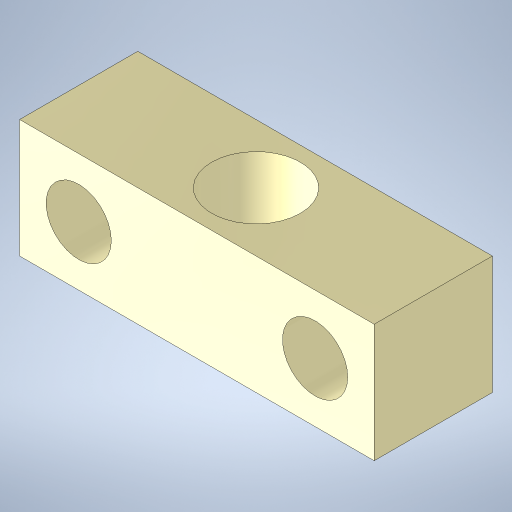
# Autodesk Inventor part: End Bushing
Saved by Autodesk Inventor 2023.2 (Build 272271000, 271)
## iProperties
Created: 2024-02-24
Part Number: End Bushing
Material: Nylon 6/6
Document SubType Name: Modeling
Designer: Nathan Cai
Density: 1.13 g/cm^3
Appearance: Nylon 6
Author: Nathan Cai
Autodesk Inventor part; units mm, degrees
ref_plane "YZ Plane" through (0, 0, 0) normal (1, 0, 0) x (0, 1, 0)
ref_plane "XZ Plane" through (0, 0, 0) normal (0, 1, 0) x (-1, 0, 0)
ref_plane "XY Plane" through (0, 0, 0) normal (0, 0, 1) x (1, 0, 0)
sketch "Sketch1" plane through (0, 0, 0) normal (0, 0, 1) x (1, 0, 0)
  line L0 (-9.525, -3.175) -> (9.525, -3.175)
  line L1 (9.525, -3.175) -> (9.525, 3.175)
  line L2 (9.525, 3.175) -> (-9.525, 3.175)
  line L3 (-9.525, 3.175) -> (-9.525, -3.175)
  line L4 (-9.525, -3.175) -> (9.525, 3.175) construction
  line L5 (9.525, -3.175) -> (-9.525, 3.175) construction
  line L6 (-3.175, -3.175) -> (3.175, -3.175)
  line L7 (3.175, -3.175) -> (3.175, 3.175)
  line L8 (3.175, 3.175) -> (-3.175, 3.175)
  line L9 (-3.175, 3.175) -> (-3.175, -3.175)
  line L10 (-3.175, -3.175) -> (3.175, 3.175) construction
  line L11 (3.175, -3.175) -> (-3.175, 3.175) construction
  line L12 (-6.35, 3.175) -> (-6.35, -3.175) construction
  line L13 (0, 3.175) -> (0, -3.175) construction
  circle A0 centre (-6.35, 0) radius 1.7526
  circle A1 centre (6.35, 0) radius 1.7526
  point P0 (0, 0)
  dimension "d0" = 19.05
  dimension "d1" = 6.35
  dimension "d2" = 6.35
  dimension "d3" = 3.175
  dimension "d4" = 3.5052
  constraints: 28 end point, 7 midpoint, 4 parallel, 3 perpendicular, 3 point on line, 2 centre point, 2 horizontal, 1 symmetric about line, 1 other
  measures "d0" distance of L2.end L1.end
  measures "d1" distance of L1.end L0.end
  measures "d2" distance of L8.end L7.end
  measures "d3" distance between parallel lines of L3 L12
  measures "d4" diameter of A0
extrude "Extrusion1" add sketch "Sketch1" along normal blind 6.35
sketch "Sketch2" plane through (-9.525, -3.175, 0) normal (0, -1, 0) x (1, 0, 0)
  line L0 (0, 6.35) -> (19.05, 6.35) projected
  line L1 (9.525, 6.35) -> (9.525, 0) construction
  circle A0 centre (9.525, 3.175) radius 2.3812
  dimension "d7" = 4.7625
  constraints: 2 end point, 2 midpoint, 1 centre point, 1 vertical
  measures "d7" diameter of A0
extrude "Extrusion2" cut sketch "Sketch2" against normal through all
body "Solid1"
